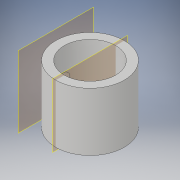
# Autodesk Inventor part: 2.2 Fuß
Saved by Autodesk Inventor 2018.3 (Build 223284000, 284)
## iProperties
Part Number: 2.2 Fuß
Material: Generisch
Document SubType Name: Modeling
Designer: pgmadmin
Density: 1 g/cm^3
Appearance: Vorgabe
Author: pgmadmin
Autodesk Inventor part; units mm, degrees
ref_plane "XZ Plane" through (0, 0, 0) normal (0, 1, 0) x (-1, 0, 0)
ref_plane "XY Plane" through (0, 0, 0) normal (0, 0, 1) x (1, 0, 0)
sketch "Skizze1" plane through (0, 0, 0) normal (0, 0, 1) x (1, 0, 0)
  circle A0 centre (0, 0) radius 10
  dimension "d0" = 20
  constraints: 1 centre point, 1 coincident
  measures "d0" diameter of A0
extrude "Extrusion1" add sketch "Skizze1" along normal blind 5
sketch "Skizze2" plane through (0, 0, 5) normal (0, 0, 1) x (1, 0, 0)
  circle A0 centre (0, 0) radius 7.5
  circle A1 centre (0, 0) radius 10
  dimension "d3" = 15
  constraints: 2 centre point, 1 coincident
  measures "d3" diameter of A0
extrude "Extrusion2" add sketch "Skizze2" along normal blind 14
sketch "Skizze3" plane through (0, 0, 0) normal (0, 0, -1) x (-1, 0, 0)
  circle A0 centre (0, 0) radius 2.45
  dimension "d6" = 4.9
  constraints: 1 centre point, 1 coincident
  measures "d6" diameter of A0
extrude "Extrusion3" cut sketch "Skizze3" against normal blind 5
ref_plane "Arbeitsebene1" through (-10, 0, 0) normal (1, 0, 0) x (0, 1, 0)
sketch "Skizze7" plane through (0, 0, 19) normal (0, 0, 1) x (1, 0, 0)
  circle A0 centre (0, 0) radius 7.5
  circle A1 centre (0, 0) radius 10
  constraints: 2 centre point, 2 coincident
extrude "Extrusion6" cut sketch "Skizze7" against normal blind 2
sketch "Skizze9" plane through (-10, 0, 0) normal (1, 0, 0) x (0, 1, 0)
  line L0 (-10, 17) -> (10, 17) projected
  line L1 (-0.2525, 8.5) -> (9.7475, 8.5)
  line L2 (-0.2525, 8.5) -> (-10.2525, 8.5)
  point P0 (0, 0)
  dimension "d36" = 8.5
  constraints: 4 end point, 2 horizontal, 1 collinear
  measures "d36" distance from line of L1.start L0
hole "Bohrung3" at (-10, -0.2525, 8.5) direction (1, 0, 0) diameter 3.5 depth 8 tip angle 118
